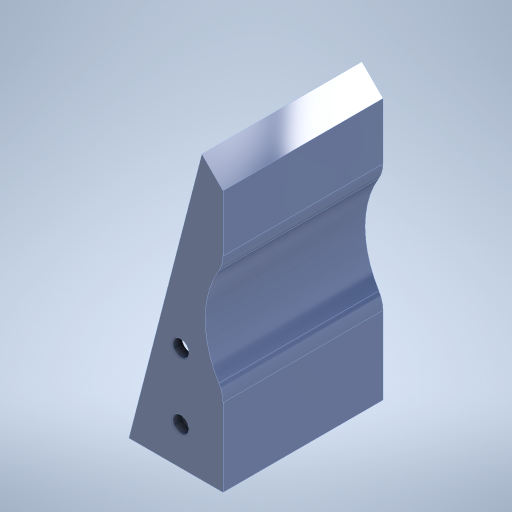
# Autodesk Inventor part: Gripper
Saved by Autodesk Inventor 2024.2 (Build 282272000, 272)
## iProperties
Created: 2025-03-19
Part Number: Gripper
Material: Generic
Document SubType Name: Modeling
Designer: migue
Density: 1 g/cm^3
Appearance: Flaked Satin - Blue
Author: migue
Autodesk Inventor part; units mm, degrees
ref_plane "YZ Plane" through (0, 0, 0) normal (1, 0, 0) x (0, 1, 0)
ref_plane "XZ Plane" through (0, 0, 0) normal (0, 1, 0) x (-1, 0, 0)
ref_plane "XY Plane" through (0, 0, 0) normal (0, 0, 1) x (1, 0, 0)
sketch "Sketch1" plane through (0, 0, 0) normal (0, 1, 0) x (-1, 0, 0)
  line L0 (0, 0) -> (-20, 0)
  line L1 (-20, 0) -> (-20, -34)
  line L2 (-20, -34) -> (0, -34)
  line L3 (0, -34) -> (0, 0)
  dimension "d0" = 34
  dimension "d1" = 20
  constraints: 8 end point, 2 parallel, 1 horizontal, 1 perpendicular
  measures "d0" distance of L2.end L0.start
  measures "d1" distance of L0.start L0.end
extrude "Extrusion1" add sketch "Sketch1" along normal blind 60
chamfer "Chamfer1" distance 4.5 angle 45 1 edges at (20, 60, -17)
sketch "Sketch3" plane through (0, 0, 0) normal (0, 0, 1) x (1, 0, 0)
  line L0 (0, 60) -> (15.5, 60) projected
  line L1 (15.5, 60) -> (0, 0)
  line L2 (0, 0) -> (20, 0) projected
  line L3 (20, 0) -> (0, 0)
  line L4 (0, 0) -> (0, 60)
  line L5 (0, 60) -> (20, 60)
  line L6 (20, 60) -> (20, 0)
  constraints: 10 end point, 2 parallel, 1 horizontal, 1 perpendicular
extrude "Extrusion2" cut sketch "Sketch3" against normal blind 60 contours L0 L1 L4
sketch "Sketch4" plane through (20, 0, -34) normal (0, 0, -1) x (-1, 0, 0)
  circle A0 centre (-16, 30) radius 19.8
  line L0 (0, 0) -> (0, 55.5) projected
  line L1 (20, 0) -> (0, 0) projected
  dimension "d9" = 39.6
  dimension "d14" = 16
  dimension "d15" = 30
  constraints: 1 centre point
  measures "d9" diameter of A0
  measures "d14" distance from line of L0 A0.centre
  measures "d15" distance from line of L1 A0.centre
extrude "Extrusion3" cut sketch "Sketch4" against normal blind 60
fillet "Fillet1" radius 6 2 edges at (20, 41.6636, -17) (20, 18.3364, -17)
shell "Shell1" thickness 2 removed faces 1 at (10.3333, 40, -22.6667)
sketch "Sketch5" plane through (0, 0, 0) normal (0, 0, 1) x (1, 0, 0)
  line L0 (0, 0) -> (20, 0) projected
  line L1 (20, 0) -> (-6.4586, 0)
  line L2 (-6.4586, 0) -> (-6.4586, 3)
  line L3 (-6.4586, 3) -> (20, 3)
  line L4 (20, 3) -> (20, 0)
  line L5 (0, 0) -> (0.775, 3)
  line L6 (15.5, 60) -> (0, 0) projected
  dimension "d16" = 3
  constraints: 10 end point, 2 parallel, 2 point on line, 1 horizontal, 1 perpendicular
  measures "d16" distance between parallel lines of L0 L3
extrude "Extrusion4" add sketch "Sketch5" against normal blind 34 contours L5 L3 L4 L0
sketch "Sketch6" plane through (0, 0, 0) normal (0, -1, 0) x (1, 0, 0)
  circle A0 centre (5, -4.5) radius 2.25
  line L0 (0, 0) -> (20, 0) projected
  line L1 (0, -34) -> (0, 0) projected
  circle A1 centre (15, -4.5) radius 2.25
  circle A2 centre (5, -29.5) radius 2.25
  circle A3 centre (15, -29.5) radius 2.25
  dimension "d19" = 4.5
  dimension "d20" = 4.5
  dimension "d21" = 5
  dimension "d24" = 10
  dimension "d27" = 25
  constraints: 4 centre point, 1 horizontal, 1 vertical, 6 other
  measures "d19" diameter of A0
  measures "d20" distance from line of L0 A0.centre
  measures "d21" distance from line of L1 A0.centre
  measures "d24" distance of A0.centre A1.centre
  measures "d27" distance of A0.centre A2.centre
extrude "Extrusion5" cut sketch "Sketch6" against normal blind 3
sketch "Sketch7" plane through (0, 0, 0) normal (0, 0, 1) x (1, 0, 0)
  circle A0 centre (11, 8) radius 1.75
  line L0 (0, 0) -> (20, 0) projected
  line L1 (20, 0) -> (20, 16.5226) projected
  line L2 (20, 0) -> (20, 15.3258)
  circle A1 centre (11, 22) radius 1.75
  dimension "d32" = 3.5
  dimension "d33" = 8
  dimension "d34" = 11
  dimension "d37" = 14
  constraints: 2 centre point, 2 end point, 1 collinear, 1 vertical, 2 other
  measures "d32" diameter of A0
  measures "d33" distance from line of L0 A0.centre
  measures "d34" horizontal distance of L0.start A0.centre
  measures "d37" distance of A0.centre A1.centre
extrude "Extrusion6" cut sketch "Sketch7" against normal through all
body "Solid1"
